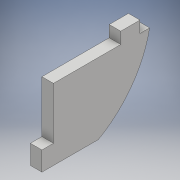
# Autodesk Inventor part: latéral
Saved by Autodesk Inventor 2017 (Build 210142000, 142)
## iProperties
Part Number: latéral
Material: Générique
Document SubType Name: Modeling
Designer: Thomas
Density: 1 g/cm^3
Appearance: Par défaut
Author: Thomas
Autodesk Inventor part; units mm, degrees
ref_plane "YZ Plane" through (0, 0, 0) normal (1, 0, 0) x (0, 1, 0)
ref_plane "XZ Plane" through (0, 0, 0) normal (0, 1, 0) x (-1, 0, 0)
ref_plane "XY Plane" through (0, 0, 0) normal (0, 0, 1) x (1, 0, 0)
sketch "Esquisse1" plane through (0, 0, 0) normal (1, 0, 0) x (0, 1, 0)
  line L0 (41, -2.0057) -> (51, -2.0057)
  line L1 (0, -45.0057) -> (0, -35.0057)
  line L2 (51, -2.0057) -> (41, -2.0057)
  line L3 (41, -2.0057) -> (41, -8.0057)
  line L4 (51, -8.0057) -> (51, -2.0057)
  line L5 (0, -35.0057) -> (6, -35.0057)
  line L6 (6, -35.0057) -> (6, -8.0057)
  line L7 (6, -45.0057) -> (0, -45.0057)
  line L8 (41, -8.0057) -> (6, -8.0057)
  line L9 (51, -8.0057) -> (56, -8.0057)
  arc A0 (29.3602, -45.0057) -> (56, -8.0057) centre (2.3964, 2.4983) ccw
  line L10 (6, -45.0057) -> (29.3602, -45.0057)
  point P0 (0, 0)
  dimension "d2" = 35
  dimension "d3" = 33
  dimension "d4" = 6
  dimension "d6" = 10
  dimension "d10" = 10
  dimension "d11" = 6
  constraints: 22 end point, 3 perpendicular, 2 horizontal, 2 point on circle, 1 centre point, 1 parallel, 1 point on line
  measures "d2" distance between parallel lines of L6 L3
  measures "d3" distance between parallel lines of L5 L0
  measures "d4" distance between parallel lines of L1 L6
  measures "d6" distance between parallel lines of L7 L5
  measures "d10" distance of L0.start L0.end
  measures "d11" distance of L4.start L0.end
extrude "Extrusion1" add sketch "Esquisse1" along normal blind 6
